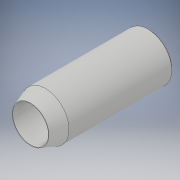
# Autodesk Inventor part: douille
Saved by Autodesk Inventor 2019 (Build 230136000, 136)
## iProperties
Created: 2019-03-25
Part Number: douille
Material: Générique
Document SubType Name: Modeling
Designer: theor
Density: 1 g/cm^3
Appearance: Par défaut
Author: theor
Autodesk Inventor part; units mm, degrees
ref_plane "YZ Plane" through (0, 0, 0) normal (1, 0, 0) x (0, 1, 0)
ref_plane "XZ Plane" through (0, 0, 0) normal (0, 1, 0) x (-1, 0, 0)
ref_plane "XY Plane" through (0, 0, 0) normal (0, 0, 1) x (1, 0, 0)
sketch "Esquisse1" plane through (0, 0, 0) normal (1, 0, 0) x (0, 1, 0)
  line L0 (0, 0) -> (0, -21.1525)
  line L1 (6, 0) -> (6, -40)
  line L2 (6.2, 0) -> (8, -4.9455)
  line L3 (8, -4.9455) -> (8, -40)
  line L4 (6, -40) -> (8, -40)
  line L5 (6, 0) -> (6.2, 0)
  dimension "d0" = 160
  dimension "d2" = 16
  dimension "d4" = 40
  dimension "d6" = 2
  dimension "d7" = 0.2
  constraints: 12 end point, 3 vertical, 2 horizontal, 1 horizontal alignment
  measures "d0" angle of L3 L2
  measures "d2" diameter of L3 L0
  measures "d4" distance from line of L1.start L4
  measures "d6" distance between parallel lines of L3 L1
  measures "d7" distance of L1.start L2.start
revolve "Révolution1" add sketch "Esquisse1" angle 360 about axis through (0, 0, 0) along (0, 0, -1)
chamfer "Chanfrein1" distance 0.5 angle 45 2 edges at (0, -6, -40) (0, -8, -40)
